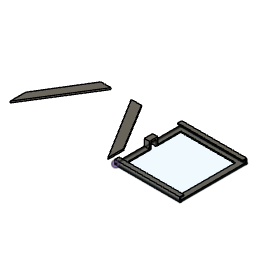
Antenna stand v2 (Autodesk Fusion 360 design; units mm, degrees)
Autodesk Fusion 360 part; units mm, degrees
sketch "Sketch1" plane through (0, 0, 0) normal (0, 0, 1) x (1, 0, 0)
  line L0 (0, 0) -> (126.3, 0)
  line L1 (126.3, 0) -> (126.3, 126.2)
  line L2 (126.3, 126.2) -> (0, 126.2)
  line L3 (0, 126.2) -> (0, 0)
  line L4 (0, 0) -> (126.3, 0)
  line L5 (126.3, 0) -> (126.3, 126.2)
  line L6 (126.3, 126.2) -> (0, 126.2)
  line L7 (0, 126.2) -> (0, 0)
  line L8 (126.3, 128.2) -> (0, 128.2)
  line L9 (0, -2) -> (126.3, -2)
  line L10 (0, 126.2) -> (0, 128.2)
  line L11 (126.3, 126.2) -> (126.3, 128.2)
  line L12 (126.3, -2) -> (126.3, 0)
  line L13 (0, 0) -> (0, -2)
  dimension "d1" = 126.3
  dimension "d2" = 126.2
  constraint horizontal L0
  constraint vertical L1
  constraint horizontal L2
  constraint vertical L3
  constraint coincident L0.start L3.end
  constraint horizontal L4
  constraint vertical L5
  constraint horizontal L6
  constraint vertical L7
  constraint perpendicular L8 L10
  constraint perpendicular L8 L11
  constraint perpendicular L4 L12
  constraint perpendicular L9 L13
  measures "d1" distance of L0.start L0.end
  measures "d2" distance of L0 L2
sketch "Sketch2" plane through (0, 0, 0) normal (0, 0, 1) x (1, 0, 0)
  line L0 (10, 10) -> (116.3, 10)
  line L1 (116.3, 10) -> (116.3, 116.3)
  line L2 (116.3, 116.3) -> (10, 116.3)
  line L3 (10, 116.3) -> (10, 10)
  dimension "d4" = 106.3
  dimension "d5" = 106.3
  constraint horizontal L0
  constraint vertical L1
  constraint horizontal L2
  constraint vertical L3
  measures "d4" distance of L0.start L0.end
  measures "d5" distance of L0.start L2.end
extrude "Extrude1" add sketch "Sketch1" along normal blind 2 makes body 1
extrude "Extrude2" cut sketch "Sketch2" along normal blind 2 bodies 1
sketch "Sketch3" plane through (0, 0, 2) normal (0, 0, 1) x (-1, 0, 0)
  line L0 (-10, -116.3) -> (-116.3, -116.3)
  line L1 (-116.3, -116.3) -> (-116.3, -10)
  line L2 (-116.3, -10) -> (-10, -10)
  line L3 (-10, -10) -> (-10, -116.3)
  line L4 (0, -128.2) -> (0, 2)
  line L5 (0, 2) -> (-126.3, 2)
  line L6 (-126.3, 2) -> (-126.3, -128.2)
  line L7 (-126.3, -128.2) -> (0, -128.2)
  line L8 (0, 0) -> (-126.3, 0)
  line L9 (-126.3, 2) -> (0, 2)
  line L10 (0, -128.2) -> (-126.3, -128.2)
  line L11 (-126.3, -128.2) -> (-126.3, -126.2)
  line L12 (-126.3, -126.2) -> (0, -126.2)
  line L13 (0, -126.2) -> (0, -128.2)
  dimension "d10" = 2
  constraint coincident L8.start origin
  constraint coincident L6 L8.end
  constraint perpendicular L6 L8
  constraint coincident L5.end L6.start
  constraint coincident L4.end L5.start
  constraint horizontal L10
  constraint vertical L11
  constraint horizontal L12
  constraint vertical L13
  constraint coincident L4.start L7.end
  measures "d10" distance of L4.start L12.end
extrude "Extrude3" add sketch "Sketch3" along normal blind 6.5 contours L4 L6 L7 L10 L11 L12 L13 | L4 L5 L6 L8 L9 bodies 1
sketch "Sketch4" plane through (0, 126.2, 0) normal (0, -1, 0) x (1, 0, 0)
  line L0 (0, 2) -> (126.3, 2)
  line L1 (126.3, 2) -> (126.3, 8.5)
  line L2 (126.3, 8.5) -> (0, 8.5)
  line L3 (0, 8.5) -> (0, 2)
  line L4 (0, 8.5) -> (126.3, 8.5)
  line L5 (126.3, 8.5) -> (126.3, 6.5)
  line L6 (126.3, 6.5) -> (0, 6.5)
  line L7 (0, 6.5) -> (0, 8.5)
  dimension "d13" = 2
  constraint horizontal L4
  constraint vertical L5
  constraint horizontal L6
  constraint vertical L7
  constraint coincident L2.end L3.start
  measures "d13" distance of L2.end L6.end
sketch "Sketch5" plane through (0, 0, 0) normal (0, 1, 0) x (-1, 0, 0)
  line L0 (-126.3, 2) -> (0, 2)
  line L1 (0, 2) -> (0, 8.5)
  line L2 (0, 8.5) -> (-126.3, 8.5)
  line L3 (-126.3, 8.5) -> (-126.3, 2)
  line L4 (-126.3, 8.5) -> (0, 8.5)
  line L5 (0, 8.5) -> (0, 6.5)
  line L6 (0, 6.5) -> (-126.3, 6.5)
  line L7 (-126.3, 6.5) -> (-126.3, 8.5)
  dimension "d14" = 2
  constraint horizontal L4
  constraint vertical L5
  constraint horizontal L6
  constraint vertical L7
  constraint coincident L2.end L3.start
  measures "d14" distance of L2.end L6.end
extrude "Extrude4" add sketch "Sketch4" along normal blind 6 contours L1 L2 L3 L4 L5 L6 L7 bodies 1
extrude "Extrude5" add sketch "Sketch5" along normal blind 6 contours L1 L2 L3 L4 L5 L6 L7 bodies 1
sketch "Sketch7" plane through (0, 0, 0) normal (0, 0, 1) x (1, 0, 0)
  line L0 (-15, 0) -> (-15, 30)
  line L1 (-15, 30) -> (-15, 0)
  line L2 (-15, 0) -> (-90.2485, 120.4228)
  line L3 (-15, 30) -> (-70.5593, 120.4228)
  line L4 (-70.5593, 120.4228) -> (-90.2485, 120.4228)
  dimension "d26" = 32
  dimension "d27" = 142
  constraint vertical L0
  constraint horizontal L4
  measures "d26" angle of L1 L2
  measures "d27" distance of L0.start L2.end
ref_plane "WorkPlane2" through (-110, 0, 0) normal (1, 0, 0) x (0, 1, 0)
extrude "Extrude7" add sketch "Sketch7" along normal blind 3 separate body makes body 2
mirror "Mirror2" about plane through (-110, 0, 0) normal (1, 0, 0) of "Extrude7" makes body 3
sketch "Sketch8" plane through (0, 0, 2) normal (0, 0, 1) x (-1, 0, 0)
  line L0 (0, 0) -> (-126.3, 0)
  line L1 (-126.3, 0) -> (-126.3, -126.2)
  line L2 (-126.3, -126.2) -> (0, -126.2)
  line L3 (0, -126.2) -> (0, 0)
  line L4 (-10, -116.3) -> (-116.3, -116.3)
  line L5 (-116.3, -116.3) -> (-116.3, -10)
  line L6 (-116.3, -10) -> (-10, -10)
  line L7 (-10, -10) -> (-10, -116.3)
  line L8 (0, -121) -> (0, -6)
  line L9 (0, -6) -> (0, -58.5)
  line L10 (0, -58.5) -> (-10, -58.5)
  line L11 (-10, -58.5) -> (-10, -68.5)
  line L12 (-10, -68.5) -> (0, -68.5)
  line L13 (0, -68.5) -> (0, -58.5)
  line L14 (0, -68.5) -> (-10, -68.5)
  line L15 (-10, -68.5) -> (-10, -71.5)
  line L16 (-10, -71.5) -> (0, -71.5)
  line L17 (0, -71.5) -> (0, -68.5)
  line L18 (0, -58.5) -> (-10, -58.5)
  line L19 (-10, -58.5) -> (-10, -55.5)
  line L20 (-10, -55.5) -> (0, -55.5)
  line L21 (0, -55.5) -> (0, -58.5)
  dimension "d33" = 52.5
  dimension "d34" = 10
  dimension "d35" = 3
  dimension "d36" = 3
  constraint coincident L3 L8.start
  constraint coincident L3 L8.end
  constraint parallel L8 L9
  constraint horizontal L10
  constraint vertical L11
  constraint horizontal L12
  constraint vertical L13
  constraint horizontal L14
  constraint vertical L15
  constraint horizontal L16
  constraint vertical L17
  constraint horizontal L18
  constraint vertical L19
  constraint horizontal L20
  constraint vertical L21
  measures "d33" distance of L8.end L9.end
  measures "d34" distance of L9.end L12.end
  measures "d35" distance of L12.end L16.end
  measures "d36" distance of L9.end L20.end
sketch "Sketch9" plane through (0, 0, 2) normal (0, 0, 1) x (-1, 0, 0)
extrude "Extrude8" add sketch "Sketch8" along normal blind 10 contours L3 L7 L8 L9 L10 L18 L19 L20 L21 | L3 L7 L8 L12 L14 L15 L16 L17 bodies 1
sketch "Sketch10" plane through (0, 0, 12) normal (0, 0, 1) x (-1, 0, 0)
  line L0 (0, -71.5) -> (0, -68.5)
  line L1 (0, -68.5) -> (-10, -68.5)
  line L2 (-10, -68.5) -> (-10, -71.5)
  line L3 (-10, -71.5) -> (0, -71.5)
  line L4 (0, -71.5) -> (-10, -71.5)
  line L5 (-10, -71.5) -> (-10, -55.5)
  line L6 (-10, -55.5) -> (0, -55.5)
  line L7 (0, -55.5) -> (0, -71.5)
  constraint horizontal L4
  constraint vertical L5
  constraint horizontal L6
  constraint vertical L7
  constraint coincident L0.start L3.end
extrude "Extrude9" add sketch "Sketch10" along normal blind 3 bodies 1
extrude "Extrude10" cut 1 faces at (3.3333, 65.1667, 2) along direction (0, 0, -1) blind 3 on bodies 1 bodies 1
